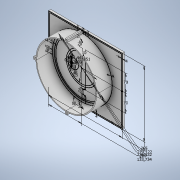
# Autodesk Inventor part: Деталь1
Saved by Autodesk Inventor 2022 (Build 260153000, 153)
## iProperties
Created: 2022-06-22
Part Number: Деталь1
Material: Типовые
Document SubType Name: Modeling
Designer: Admin
Density: 1 g/cm^3
Appearance: По умолчанию
Author: Admin
Autodesk Inventor part; units mm, degrees
ref_plane "YZ Plane" through (0, 0, 0) normal (1, 0, 0) x (0, 1, 0)
ref_plane "XZ Plane" through (0, 0, 0) normal (0, 1, 0) x (-1, 0, 0)
ref_plane "XY Plane" through (0, 0, 0) normal (0, 0, 1) x (1, 0, 0)
sketch "Эскиз1" plane through (0, 0, 0) normal (0, 0, 1) x (1, 0, 0)
  line L0 (-133.734, -132.5) -> (163.266, -132.5)
  line L1 (163.266, -132.5) -> (163.266, 132.5)
  line L2 (163.266, 132.5) -> (-133.734, 132.5)
  line L3 (-133.734, 132.5) -> (-133.734, -132.5)
  circle A0 centre (0, 0) radius 104.5
  line L4 (159.266, 128.5) -> (159.266, -128.5)
  circle A1 centre (0, 0) radius 110.061
  circle A2 centre (0, 0) radius 118.266
  line L5 (5, -122.1637) -> (5, -130.5)
  line L6 (5, -130.5) -> (-5, -130.5)
  line L7 (-5, -130.5) -> (-5, -122.1637)
  line L8 (159.266, -128.5) -> (5, -128.5)
  line L9 (-5, -128.5) -> (-129.734, -128.5)
  line L10 (5, 122.1637) -> (5, 130.5)
  line L11 (5, 130.5) -> (-5, 130.5)
  line L12 (-5, 130.5) -> (-5, 122.1637)
  arc A3 (5, -122.1637) -> (5, 122.1637) centre (0, 0) ccw
  arc A4 (-45.941, -17.5) -> (-38.941, -17.5) centre (-42.441, -17.5) ccw
  circle A5 centre (-42.441, -17.5) radius 2
  circle A6 centre (-34.441, 0) radius 2.5 construction
  line L13 (-38.941, -17.5) -> (-38.941, 17.5)
  line L14 (-42.441, 17.5) -> (-42.441, -17.5)
  line L15 (-45.941, 17.5) -> (-45.941, -17.5)
  circle A7 centre (-42.441, 17.5) radius 2
  circle A8 centre (-34.441, 0) radius 20.7845
  arc A9 (-38.941, 17.5) -> (-45.941, 17.5) centre (-42.441, 17.5) ccw
  circle A10 centre (0, 0) radius 62
  circle A11 centre (0, 0) radius 55.4255
  line L16 (12.766, 90) -> (6.766, 90)
  line L17 (4.766, 88) -> (4.766, 72)
  line L18 (6.766, 70) -> (12.766, 70)
  line L19 (12.766, -70) -> (6.766, -70)
  line L20 (4.766, -72) -> (4.766, -88)
  line L21 (6.766, -90) -> (12.766, -90)
  line L22 (14.766, 132.5) -> (14.766, 92)
  line L23 (14.766, 68) -> (14.766, -68)
  line L24 (14.766, -92) -> (14.766, -132.5)
  arc A12 (6.766, 90) -> (4.766, 88) centre (6.766, 88) ccw
  arc A13 (4.766, 72) -> (6.766, 70) centre (6.766, 72) ccw
  arc A14 (4.766, -88) -> (6.766, -90) centre (6.766, -88) ccw
  arc A15 (6.766, -70) -> (4.766, -72) centre (6.766, -72) ccw
  arc A16 (12.766, -70) -> (14.766, -68) centre (12.766, -68) ccw
  arc A17 (14.766, -92) -> (12.766, -90) centre (12.766, -92) ccw
  arc A18 (14.766, 68) -> (12.766, 70) centre (12.766, 68) ccw
  arc A19 (12.766, 90) -> (14.766, 92) centre (12.766, 92) ccw
  line L25 (-129.734, 128.5) -> (-5, 128.5)
  line L26 (5, 128.5) -> (159.266, 128.5)
  line L27 (0, 130.5) -> (0, 118.266)
  line L28 (0, -118.266) -> (0, -130.5)
  line L29 (122.266, 0) -> (118.266, 0)
  line L30 (-122.1637, 5) -> (-131.734, 5)
  line L31 (-131.734, 5) -> (-131.734, -5)
  line L32 (-131.734, -5) -> (-122.1637, -5)
  arc A20 (-5, 122.1637) -> (-122.1637, 5) centre (0, 0) ccw
  arc A21 (-122.1637, -5) -> (-5, -122.1637) centre (0, 0) ccw
  line L33 (118.266, 0) -> (122.266, 0)
  line L34 (-129.734, -128.5) -> (-129.734, -5)
  line L35 (-129.734, 5) -> (-129.734, 128.5)
  line L36 (-131.734, 0) -> (-118.266, 0)
  point P0 (163.266, 0)
  point P1 (5, -126.3319)
  point P2 (-5, -126.3319)
  point P3 (-42.441, -21)
  point P4 (-38.941, 0)
  point P5 (-45.941, 0)
  point P6 (-55.2255, 0)
  point P7 (-42.441, 21)
  point P8 (-55.4255, 0)
  point P9 (4.766, 70)
  point P10 (4.766, 90)
  point P11 (14.766, 70)
  point P12 (4.766, -90)
  point P13 (4.766, -70)
  point P14 (14.766, -90)
  point P15 (14.766, 128.5)
  point P16 (14.766, -128.5)
  point P17 (14.766, -117.3406)
  point P18 (14.766, 117.3406)
  point P19 (14.766, 121.3711)
  dimension "d19" = 41.569
  dimension "d20" = 110.851
  dimension "d0" = 265
  dimension "d1" = 297
  dimension "d2" = 209
  dimension "d3" = 220.122
  dimension "d4" = 236.532
  dimension "d5" = 133.734
  dimension "d6" = 10
  dimension "d7" = 4
  dimension "d8" = 4
  dimension "d9" = 2
  dimension "d10" = 10
  dimension "d11" = 2
  dimension "d12" = 4
  dimension "d13" = 124
  dimension "d14" = 35
  dimension "d15" = 3.5
  dimension "d16" = 4
  dimension "d17" = 4
  dimension "d18" = 5
  dimension "d21" = 0.2
  dimension "d22" = 4.5
  dimension "d23" = 42.441
  dimension "d24" = 10
  dimension "d25" = 20
  dimension "d26" = 10
  dimension "d27" = 20
  dimension "d28" = 70
  dimension "d29" = 70
  dimension "d30" = 2
  dimension "d31" = 4
  dimension "d32" = 4
  dimension "d33" = 4
  dimension "d34" = 2
  dimension "d35" = 10
  dimension "d36" = 4
  dimension "d37" = 4
  dimension "d38" = 4
  constraints: 74 end point, 33 point on circle, 20 centre point, 20 tangent, 19 point on line, 17 coincident, 14 horizontal alignment, 14 parallel, 12 perpendicular, 11 midpoint, 8 vertical alignment, 7 equal radius, 5 vertical, 4 horizontal, 1 collinear, 4 other
  measures "d0" distance of L0.end L2.start
  measures "d1" distance of L0.start L0.end
  measures "d2" diameter of A0
  measures "d3" diameter of A1
  measures "d4" diameter of A2
  measures "d5" distance from line of L3 point (0, 0)
  measures "d6" distance between parallel lines of L7 L5
  measures "d7" distance between parallel lines of L0 L8
  measures "d8" distance between parallel lines of L0 L9
  measures "d9" distance between parallel lines of L0 L6
  measures "d10" distance between parallel lines of L12 L10
  measures "d11" distance between parallel lines of L2 L11
  measures "d12" radial gap between concentric circles of A2 A3
  measures "d13" diameter of A10
  measures "d14" distance of L15.end L15.start
  measures "d15" radius of A9
  measures "d16" diameter of A5
  measures "d17" diameter of A7
  measures "d18" diameter of A6
  measures "d21" distance of point (-55.426, 0) point (-55.226, 0)
  measures "d22" distance from line of L13 A6.centre
  measures "d23" distance from line of point (0, 0) L14
  measures "d24" distance of point (14.766, 70) point (4.766, 70)
  measures "d25" distance of point (4.766, 70) point (4.766, 90)
  measures "d26" distance of point (14.766, -90) point (4.766, -90)
  measures "d27" distance of point (4.766, -90) point (4.766, -70)
  measures "d28" distance from line of A1.centre L19
  measures "d29" distance from line of point (0, 0) L18
  measures "d30" radius of A12
  measures "d31" distance between parallel lines of L2 L26
  measures "d32" distance between parallel lines of L2 L25
  measures "d33" distance between parallel lines of L1 L4
  measures "d34" distance between parallel lines of L3 L31
  measures "d35" distance between parallel lines of L30 L32
  measures "d36" radial gap between concentric circles of A2 A20
  measures "d37" distance between parallel lines of L3 L35
  measures "d38" distance between parallel lines of L3 L34
extrude "Выдавливание1" add sketch "Эскиз1" against normal blind 9 contours L3 L2 L22 L26 L10 L11 L12 L25 L35 L30 L31 L32 L34 L9 L7 L6 L5 L8 L24 L0 | L8 L5 A3 L24 | L5 L6 L28 A2 L24 A3 | L22 A3 L10 L26 | A2 L22 A1 L24 | L22 A2 L27 L11 L10 A3 | L6 L7 A21 L32 L31 L36 A2 L28 | A1 L22 A0 L24 | L36 L31 L30 A20 L12 L11 L27 A2 | A0 L22 A19 L16 A12 L17 A13 L18 A18 L23 A10 A16 L19 A15 L20 A14 L21 A17 L24 | L9 L34 L32 A21 L7 | L12 A20 L30 L35 L25 | A10 L23 A11 | A11 L23 | L15 A8 A5 A4 | A8 A5 L14 A7 A9 L13 A4 | A4 L13 A9 A8 | A8 L15 | L15 A8 A7 L14 A5 | A8 A5 | A5 A8 | L15 A9 A8 A7 | A8 A7 | A7 A8 picked at (-84.4797, -74.5018) picked at (-106.1903, 0) picked at (-8.6565, -83.7412) picked at (-12.9584, 58.1755) picked at (5.2918, 0)
extrude "Выдавливание2" add sketch "Эскиз1" against normal blind 9 separate body contours L24 L8 L4 L26 L22 L2 L1 L0 | L24 A3 L22 L26 L4 L8 | L24 A2 L29 A3 | L29 A2 L22 A3 | L24 A1 L22 A2 | L24 A0 L22 A1 | L24 A17 L21 A14 L20 A15 L19 A16 L23 A10 A18 L18 A13 L17 A12 L16 A19 L22 A0 | L23 A11 A10 | L23 A11 picked at (84.701, 74.2521) picked at (107.6015, -9.289) picked at (74.2357, -51.1207) picked at (38.5792, -42.5793) picked at (20.8983, 14.8032)
extrude "Выдавливание4" cut sketch "Эскиз1" against normal blind 2 contours L5 L6 L28 A2 L24 A3 | L24 A2 L29 A3 | L29 A2 L22 A3 | L22 A2 L27 L11 L10 A3 | L6 L7 A21 L32 L31 L36 A2 L28 | L36 L31 L30 A20 L12 L11 L27 A2 bodies 2 1
extrude "Выдавливание5" cut sketch "Эскиз1" against normal blind 1.5 contours L24 A0 L22 A1 | A1 L22 A0 L24 bodies 2 1
extrude "Выдавливание6" add sketch "Эскиз1" along normal blind 62 and the other way blind 2 separate body contours L6 L7 A21 L32 L31 L36 A2 L28
extrude "Выдавливание7" add sketch "Эскиз1" along normal blind 62 and the other way blind 2 separate body contours L5 L6 L28 A2 L24 A3 | L24 A2 L29 A3
extrude "Выдавливание8" add sketch "Эскиз1" along normal blind 62 and the other way blind 2 separate body contours L29 A2 L22 A3 | L22 A2 L27 L11 L10 A3
extrude "Выдавливание9" add sketch "Эскиз1" along normal blind 62 and the other way blind 2 separate body contours L36 L31 L30 A20 L12 L11 L27 A2
sketch "Эскиз2" plane through (14.766, -132.5, 0) normal (0, -1, 0) x (1, 0, 0)
  line L0 (0, 0) -> (148.5, 0) projected
  circle A0 centre (108.5, 0) radius 5
  line L1 (-148.5, 0) -> (0, 0) projected
  circle A1 centre (-108.5, 0) radius 5
  line L2 (0, 0) -> (0, -9) construction
  line L3 (0, 0) -> (0, -9) construction
  line L4 (0, 0) -> (0, -9) projected
  line L5 (-148.5, 0) -> (-148.5, -9) projected
  line L6 (148.5, 0) -> (148.5, -9) projected
  line L7 (148.5, 0) -> (148.5, 36)
  line L8 (148.5, 36) -> (118.5, 66)
  line L9 (118.5, 66) -> (-148.5, 66)
  line L10 (-148.5, 66) -> (-148.5, 0)
  line L11 (-148.5, 62) -> (116.8431, 62)
  line L12 (116.8431, 62) -> (144.5, 34.3431)
  line L13 (144.5, 34.3431) -> (144.5, 0)
  line L14 (144.5, 34.3431) -> (148.5, 36)
  line L15 (118.5, 66) -> (116.8431, 62)
  circle A2 centre (130.6716, 48.1716) radius 2
  circle A3 centre (144.5, 17.1716) radius 2
  point P0 (-14.766, 0)
  point P1 (107.5, 62)
  dimension "d43" = 10
  dimension "d44" = 10
  dimension "d45" = 40
  dimension "d68" = 30
  dimension "d69" = 30
  dimension "d70" = 4
  dimension "d71" = 4
  dimension "d72" = 4
  dimension "d73" = 4
  dimension "d74" = 4
  constraints: 20 end point, 6 point on line, 4 centre point, 3 perpendicular, 2 collinear, 2 midpoint, 1 horizontal, 1 parallel, 1 symmetric about line
  measures "d43" diameter of A0
  measures "d44" diameter of A1
  measures "d45" distance from line of A1.centre L5
  measures "d68" horizontal distance of L7.end L8.end
  measures "d69" horizontal distance of L7.end L8.end
  measures "d70" distance between parallel lines of L9 L11
  measures "d71" distance between parallel lines of L8 L12
  measures "d72" distance between parallel lines of L7 L13
  measures "d73" diameter of A2
  measures "d74" diameter of A3
extrude "Выдавливание3" cut sketch "Эскиз2" against normal blind 6 contours A0 L0 | L0 A0 | A1 L1 | L1 A1 bodies 2 1
